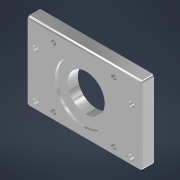
# Autodesk Inventor part: MONTURA DE MOTOR DE ELEVACIÓN
Saved by Autodesk Inventor 2022 (Build 260153000, 153)
## iProperties
Created: 2021-09-22
Part Number: MONTURA DE MOTOR DE ELEVACIÓN
Material: Aluminum 6061
Document SubType Name: Modeling
Designer: Andres
Density: 2.7 g/cm^3
Appearance: Aluminum - Flat
Mass: 120.448 g
Surface Area: 141.93 cm^2
Volume: 44.6102 cm^3
Author: Andres
Autodesk Inventor part; units mm, degrees
ref_plane "YZ Plane" through (0, 0, 0) normal (1, 0, 0) x (0, 1, 0)
ref_plane "XZ Plane" through (0, 0, 0) normal (0, 1, 0) x (-1, 0, 0)
ref_plane "XY Plane" through (0, 0, 0) normal (0, 0, 1) x (1, 0, 0)
sketch "Sketch1" plane through (0, 0, 0) normal (0, 0, 1) x (1, 0, 0)
  line L0 (3, 10) -> (25, 10) projected
  line L1 (115, 10) -> (137, 10) projected
  circle A0 centre (70, -10) radius 14.5
  arc A1 (113, -40) -> (115, -38) centre (113, -38) ccw projected
  line L2 (113, -40) -> (27, -40) projected
  arc A2 (25, -38) -> (27, -40) centre (27, -38) ccw projected
  line L3 (115, 10) -> (115, -38) projected
  line L4 (25, -38) -> (25, 10) projected
  line L5 (25, 10) -> (25, 21)
  line L6 (25, 21) -> (115, 21)
  line L7 (115, 21) -> (115, 10)
  line L8 (3, -42) -> (3, 10) projected
  line L9 (137, 10) -> (137, -42) projected
  circle A3 centre (125, -33.5) radius 1.621 projected
  circle A4 centre (15, -1.5) radius 1.621 projected
  circle A5 centre (15, -33.5) radius 1.621 projected
  circle A6 centre (125, -1.5) radius 1.621 projected
  circle A7 centre (70, -10) radius 12.5 projected
  line L10 (137, -42) -> (3, -42) projected
  dimension "d6" = 31
  dimension "d7" = 30
  dimension "d39" = 2
  constraints: 6 end point, 2 perpendicular, 1 centre point, 1 concentric, 1 vertical
  measures "d6" distance from line of A0.centre L6
  measures "d7" distance from line of L2 A0.centre
  measures "d39" radial gap between concentric circles of A0 A7
extrude "Extrusion1" add sketch "Sketch1" along normal mid plane 8 contours L5 L6 L7 L3 A1 L2 A2 L4
sketch "Sketch6" plane through (0, 0, 4) normal (0, 0, 1) x (1, 0, 0)
  circle A0 centre (70, -10) radius 14.5 projected
  circle A1 centre (70, -10) radius 22.5
  line L0 (115, 21) -> (25, 21) projected
  line L1 (25, 21) -> (25, -38) projected
  arc A2 (25, -38) -> (27, -40) centre (27, -38) ccw projected
  line L2 (27, -40) -> (113, -40) projected
  arc A3 (113, -40) -> (115, -38) centre (113, -38) ccw projected
  line L3 (115, -38) -> (115, 21) projected
  circle A4 centre (70, -10) radius 14.5 projected
  point P0 (0, 0)
  dimension "d25" = 45
  constraints: 1 centre point, 1 coincident
  measures "d25" diameter of A1
extrude "Extrusion2" add sketch "Sketch6" along normal blind 2 contours L3 A3 L2 A2 L1 L0
sketch "Sketch5" plane through (0, 0, 6) normal (0, 0, 1) x (1, 0, 0)
  circle A0 centre (46.5, 13.5) radius 3.1 projected
  circle A1 centre (46.5, -33.5) radius 3.1 projected
  circle A2 centre (93.5, -33.5) radius 3.1 projected
  circle A3 centre (93.5, 13.5) radius 3.1 projected
  point P0 (0, 0)
  point P1 (46.5, 13.5)
  point P2 (46.5, -33.5)
  point P3 (93.5, 13.5)
  point P4 (93.5, -33.5)
hole "Hole2" at (46.5, 13.5, 6) at (46.5, -33.5, 6) at (93.5, -33.5, 6) at (93.5, 13.5, 6) direction (0, 0, -1) diameter 4.134 depth 8.2 tip angle 118 thread size "M5x0.8" class "6H" standard "ISO Metric profile"
sketch "Sketch7" plane through (0, 0, 6) normal (0, 0, 1) x (1, 0, 0)
  circle A0 centre (70, -10) radius 14.5 projected
  line L0 (32.5, -34) -> (107.5, -34) construction
  line L1 (107.5, -34) -> (107.5, 2) construction
  line L2 (107.5, 2) -> (32.5, 2) construction
  line L3 (32.5, 2) -> (32.5, -34) construction
  line L4 (32.5, -34) -> (107.5, 2) construction
  line L5 (107.5, -34) -> (32.5, 2) construction
  point P0 (0, 0)
  point P1 (70, -16)
  point P2 (70, -16)
  dimension "d28" = 75
  dimension "d29" = 36
  dimension "d30" = 6
  constraints: 12 end point, 3 midpoint, 2 parallel, 1 horizontal, 1 perpendicular, 1 vertical alignment
  measures "d28" distance of L1.end L2.end
  measures "d29" distance of L2.end L0.start
  measures "d30" distance of A0.centre point (70, -16)
hole "Hole3" at (32.5, 2, 6) at (32.5, -34, 6) at (107.5, -34, 6) at (107.5, 2, 6) direction (0, 0, -1) diameter 4.5 end through all clearance for "Socket Head Cap Screw ISO 4762" size "M4" standard "ISO"
fillet "Fillet1" radius 2 8 edges at (114.4142, -39.4142, 6) (70, -40, 6) (25.5858, -39.4142, 6) (25, -8.5, 6) (115, -8.5, 6) (70, 21, 6) (115, 21, 1) (25, 21, 1)
body "Solid1"
